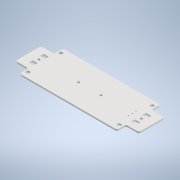
# Autodesk Inventor part: Interstage B1
Saved by Autodesk Inventor 2020.3 (Build 243373000, 373)
## iProperties
Created: 2020-05-18
Part Number: Interstage B1
Material: Genérico
Document SubType Name: Modeling
Designer: javic
Density: 1 g/cm^3
Appearance: Valor por defecto
Author: javic
Autodesk Inventor part; units mm, degrees
ref_plane "YZ Plane" through (0, 0, 0) normal (1, 0, 0) x (0, 1, 0)
ref_plane "XZ Plane" through (0, 0, 0) normal (0, 1, 0) x (-1, 0, 0)
ref_plane "XY Plane" through (0, 0, 0) normal (0, 0, 1) x (1, 0, 0)
sketch "Boceto1" plane through (0, 0, 0) normal (0, 1, 0) x (-1, 0, 0)
  arc A0 (-10.02, 7.27) -> (-8.75, 6) centre (-8.75, 7.27) ccw
  line L0 (-8.75, 6) -> (-2.54, 6)
  arc A1 (-1.27, 4.73) -> (-2.54, 6) centre (-2.54, 4.73) ccw
  line L1 (-1.27, 4.73) -> (-1.27, 1.27)
  arc A2 (-1.27, 1.27) -> (0, 0) centre (0, 1.27) ccw
  line L2 (0, 0) -> (62.46, 0)
  arc A3 (62.46, 0) -> (63.73, 1.27) centre (62.46, 1.27) ccw
  line L3 (63.73, 1.27) -> (63.73, 4.73)
  arc A4 (65, 6) -> (63.73, 4.73) centre (65, 4.73) ccw
  line L4 (65, 6) -> (71.21, 6)
  arc A5 (71.21, 6) -> (72.48, 7.27) centre (71.21, 7.27) ccw
  line L5 (72.48, 7.27) -> (72.48, 21.73)
  arc A6 (72.48, 21.73) -> (71.21, 23) centre (71.21, 21.73) ccw
  line L6 (71.21, 23) -> (65, 23)
  arc A7 (63.73, 24.27) -> (65, 23) centre (65, 24.27) ccw
  line L7 (63.73, 24.27) -> (63.73, 27.73)
  arc A8 (63.73, 27.73) -> (62.46, 29) centre (62.46, 27.73) ccw
  line L8 (62.46, 29) -> (0, 29)
  arc A9 (0, 29) -> (-1.27, 27.73) centre (0, 27.73) ccw
  line L9 (-1.27, 27.73) -> (-1.27, 24.27)
  arc A10 (-2.54, 23) -> (-1.27, 24.27) centre (-2.54, 24.27) ccw
  line L10 (-2.54, 23) -> (-8.75, 23)
  arc A11 (-8.75, 23) -> (-10.02, 21.73) centre (-8.75, 21.73) ccw
  line L11 (-10.02, 21.73) -> (-10.02, 7.27)
  circle A12 centre (61.755, 25.475) radius 1.25
  circle A13 centre (0.755, 3.475) radius 1.25
  circle A14 centre (0.755, 25.475) radius 1.25
  circle A15 centre (61.755, 3.475) radius 1.25
  circle A16 centre (38.98, 14.5) radius 0.9
  circle A17 centre (23.98, 14.5) radius 0.9
  point P0 (0, 0)
  constraints: 27 tangent, 24 end point, 24 point on circle, 18 centre point, 15 equal radius, 4 parallel, 4 perpendicular
extrude "Extrusión1" add sketch "Boceto1" along normal blind 1.04
sketch "Boceto2" plane through (0, 1.04, 0) normal (0, 1, 0) x (1, 0, 0)
  circle A0 centre (-65.48, -14.5) radius 0.9
  circle A1 centre (3.02, -14.5) radius 0.9
  line L0 (-71.21, -23) -> (-65, -23) projected
  line L1 (-72.48, -7.27) -> (-72.48, -21.73) projected
  line L2 (2.54, -23) -> (8.75, -23) projected
  line L3 (10.02, -21.73) -> (10.02, -7.27) projected
  point P0 (0, 0)
  dimension "d2" = 1.8
  dimension "d3" = 1.8
  dimension "d4" = 8.5
  dimension "d5" = 7
  dimension "d6" = 8.5
  dimension "d7" = 7
  constraints: 2 centre point
  measures "d2" diameter of A0
  measures "d3" diameter of A1
  measures "d4" distance from line of L0 A0.centre
  measures "d5" distance from line of L1 A0.centre
  measures "d6" distance from line of L2 A1.centre
  measures "d7" distance from line of L3 A1.centre
hole "Agujero1" at (-65.48, 1.04, 14.5) at (3.02, 1.04, 14.5) direction (0, -1, 0) diameter 1.8 end through all
sketch "Boceto3" plane through (0, 1.04, 0) normal (0, 1, 0) x (1, 0, 0)
  circle A0 centre (-3.08, -11.96) radius 0.4
  line L0 (0, 0) -> (-62.46, 0) projected
  line L1 (10.02, -21.73) -> (10.02, -7.27) projected
  circle A1 centre (-3.08, -14.5) radius 0.4
  circle A2 centre (-3.08, -17.04) radius 0.4
  line L2 (-62.46, -29) -> (0, -29) projected
  line L3 (1.27, -27.73) -> (1.27, -24.27) projected
  dimension "d23" = 0.8
  dimension "d24" = 11.96
  dimension "d25" = 13.1
  dimension "d26" = 0.8
  dimension "d27" = 0.8
  dimension "d28" = 13.1
  dimension "d29" = 13.1
  dimension "d30" = 11.96
  dimension "d31" = 2.54
  dimension "d32" = 2.54
  dimension "d40" = 4.35
  constraints: 3 centre point
  measures "d23" diameter of A0
  measures "d24" distance from line of L0 A0.centre
  measures "d25" distance from line of L1 A0.centre
  measures "d26" diameter of A1
  measures "d27" diameter of A2
  measures "d28" distance from line of L1 A1.centre
  measures "d29" distance from line of L1 A2.centre
  measures "d30" distance from line of L2 A2.centre
  measures "d31" distance of A1.centre A0.centre
  measures "d32" distance of A2.centre A1.centre
  measures "d40" distance from line of L3 A2.centre
hole "Agujero2" at (-3.08, 1.04, 11.96) at (-3.08, 1.04, 14.5) at (-3.08, 1.04, 17.04) direction (0, -1, 0) diameter 0.8 end through all
sketch "Boceto4" plane through (0, 0, 0) normal (0, -1, 0) x (1, 0, 0)
  line L0 (4.72, 9.6) -> (1.32, 9.6)
  line L1 (1.32, 9.6) -> (1.32, 12)
  line L2 (1.32, 12) -> (4.72, 12)
  line L3 (4.72, 12) -> (4.72, 9.6)
  line L4 (4.72, 17) -> (1.32, 17)
  line L5 (1.32, 17) -> (1.32, 19.4)
  line L6 (1.32, 19.4) -> (4.72, 19.4)
  line L7 (4.72, 19.4) -> (4.72, 17)
  line L8 (10.02, 21.73) -> (10.02, 7.27) projected
  line L9 (2.54, 23) -> (8.75, 23) projected
  line L10 (8.75, 6) -> (2.54, 6) projected
  line L11 (-63.78, 19.4) -> (-67.18, 19.4)
  line L12 (-67.18, 19.4) -> (-67.18, 17)
  line L13 (-67.18, 17) -> (-63.78, 17)
  line L14 (-63.78, 17) -> (-63.78, 19.4)
  line L15 (-71.21, 23) -> (-65, 23) projected
  line L16 (-72.48, 7.27) -> (-72.48, 21.73) projected
  line L17 (-63.78, 9.6) -> (-67.18, 9.6)
  line L18 (-67.18, 9.6) -> (-67.18, 12)
  line L19 (-67.18, 12) -> (-63.78, 12)
  line L20 (-63.78, 12) -> (-63.78, 9.6)
  line L21 (-65, 6) -> (-71.21, 6) projected
  point P0 (0, 0)
  dimension "d41" = 3.4
  dimension "d42" = 2.4
  dimension "d43" = 3.4
  dimension "d44" = 2.4
  dimension "d45" = 5.3
  dimension "d46" = 3.6
  dimension "d47" = 3.6
  dimension "d48" = 3.4
  dimension "d49" = 2.4
  dimension "d50" = 3.6
  dimension "d51" = 5.3
  dimension "d52" = 3.6
  dimension "d53" = 5.3
  constraints: 32 end point, 8 parallel, 4 horizontal, 4 perpendicular, 1 point on line
  measures "d41" distance of L1.end L2.end
  measures "d42" distance of L0.end L1.end
  measures "d43" distance of L5.end L6.end
  measures "d44" distance of L4.end L5.end
  measures "d45" distance between parallel lines of L8 L3
  measures "d46" distance between parallel lines of L9 L6
  measures "d47" distance between parallel lines of L10 L0
  measures "d48" distance of L13.end L12.end
  measures "d49" distance of L12.end L11.end
  measures "d50" distance between parallel lines of L15 L11
  measures "d51" distance between parallel lines of L16 L12
  measures "d52" distance between parallel lines of L21 L17
  measures "d53" distance between parallel lines of L16 L18
extrude "Extrusión2" cut sketch "Boceto4" against normal through all
